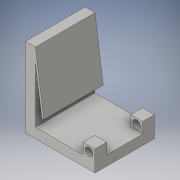
# Autodesk Inventor part: gpsFrame
Saved by Autodesk Inventor 2016 (Build 200138000, 138)
## iProperties
Created: 2016-10-13
Part Number: gpsFrame
Material: Generic
Document SubType Name: Modeling
Designer: lachesis
Density: 1 g/cm^3
Appearance: Default
Author: lachesis
Autodesk Inventor part; units mm, degrees
ref_plane "YZ Plane" through (0, 0, 0) normal (1, 0, 0) x (0, 1, 0)
ref_plane "XZ Plane" through (0, 0, 0) normal (0, 1, 0) x (-1, 0, 0)
ref_plane "XY Plane" through (0, 0, 0) normal (0, 0, 1) x (1, 0, 0)
sketch "Sketch1" plane through (0, 0, 0) normal (0, 0, 1) x (1, 0, 0)
  line L0 (0, 40) -> (5, 40)
  line L1 (5, 40) -> (5, 0)
  line L2 (5, 0) -> (0, 0)
  line L3 (0, 0) -> (0, 40)
  line L4 (5, 0) -> (35, 0)
  line L5 (35, 0) -> (35, 5)
  line L6 (35, 5) -> (5, 5)
  line L7 (5, 5) -> (5, 0)
  line L8 (35, 5) -> (29, 5)
  line L9 (29, 5) -> (29, 10.5)
  line L10 (29, 10.5) -> (35, 10.5)
  line L11 (35, 10.5) -> (35, 5)
  dimension "d0" = 5
  dimension "d1" = 5
  dimension "d2" = 30
  dimension "d4" = 35
  dimension "d7" = 5.5
  dimension "d8" = 6
  constraints: 24 end point, 6 parallel, 3 horizontal, 3 perpendicular, 1 coincident
  measures "d0" distance between parallel lines of L1 L3
  measures "d1" distance between parallel lines of L4 L6
  measures "d2" distance between parallel lines of L5 L1
  measures "d4" distance between parallel lines of L6 L0
  measures "d7" distance of L10.end L5.end
  measures "d8" distance of L9.end L10.end
extrude "Extrusion1" add sketch "Sketch1" along normal blind 30
sketch "Sketch2" plane through (0, 0, 30) normal (0, 0, 1) x (1, 0, 0)
  line L0 (35, 0) -> (35, 10.5) projected
  line L1 (35, 10.5) -> (29, 10.5) projected
  line L2 (29, 10.5) -> (29, 5) projected
  line L3 (29, 5) -> (5, 5) projected
  line L4 (5, 5) -> (5, 40) projected
  line L5 (5, 40) -> (0, 40) projected
  line L6 (0, 40) -> (0, 0) projected
  line L7 (0, 0) -> (35, 0) projected
  line L8 (5, 40) -> (9.2143, 10.5)
  line L9 (9.2143, 10.5) -> (8.2143, 10.5)
  line L10 (8.2143, 10.5) -> (5, 33)
  line L11 (5, 5) -> (5, 40) projected
  line L12 (5, 40) -> (5, 33)
  point P0 (8.7143, 10.5)
  point P1 (32, 10.5)
  dimension "d9" = 1
  dimension "d10" = 7
  constraints: 8 end point, 2 midpoint, 1 collinear, 1 horizontal, 1 horizontal alignment, 1 parallel, 1 point on line
  measures "d9" distance of L8.end L9.end
  measures "d10" distance of L4.end L10.end
extrude "Extrusion2" add sketch "Sketch2" against normal up to surface (30 mm away) contours L8 L9 L10 L4
sketch "Sketch3" plane through (0, 0, 30) normal (0, 0, 1) x (1, 0, 0)
  line L0 (35, 0) -> (35, 10.5) projected
  line L1 (35, 10.5) -> (29, 10.5) projected
  line L2 (29, 10.5) -> (29, 5) projected
  line L3 (29, 5) -> (5, 5) projected
  line L4 (5, 5) -> (5, 33) projected
  line L5 (5, 33) -> (8.2143, 10.5) projected
  line L6 (8.2143, 10.5) -> (9.2143, 10.5) projected
  line L7 (9.2143, 10.5) -> (5, 40) projected
  line L8 (5, 40) -> (0, 40) projected
  line L9 (0, 40) -> (0, 0) projected
  line L10 (0, 0) -> (35, 0) projected
  point P0 (32, 7.75)
  point P1 (29, 7.75)
  point P2 (32, 10.5)
  constraints: 2 midpoint, 1 horizontal alignment, 1 vertical alignment
hole "Hole1" at (32, 7.75, 30) direction (0, 0, -1) diameter 4 end through all
sketch "Sketch4" plane through (29, 10.5, 0) normal (0, 1, 0) x (1, 0, 0)
  line L0 (6, 0) -> (0, 0) projected
  line L1 (0, 0) -> (0, -30) projected
  line L2 (6, -30) -> (0, -30) projected
  line L3 (6, 0) -> (6, -30) projected
  line L4 (0, 0) -> (0, -30) projected
  line L5 (6, 0) -> (6, -30) projected
  line L6 (0, -6) -> (6, -6)
  line L7 (6, -6) -> (6, -24)
  line L8 (6, -24) -> (0, -24)
  line L9 (0, -24) -> (0, -6)
  point P0 (-29, 0)
  dimension "d20" = 6
  dimension "d21" = 6
  constraints: 8 end point, 2 parallel, 2 point on line, 1 horizontal, 1 perpendicular
  measures "d20" distance between parallel lines of L6 L0
  measures "d21" distance between parallel lines of L2 L8
extrude "Extrusion3" cut sketch "Sketch4" against normal up to surface (5.5 mm away) contours L3 L8 L1 L6
equation "\"d21\" = d20"
body "Solid1"
